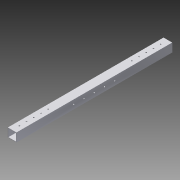
# Autodesk Inventor part: crossbar(cb)
Saved by Autodesk Inventor 2015 (Build 190159000, 159)
## iProperties
Created: 2015-10-09
Part Number: crossbar(cb)
Material: Aluminum 6061
Document SubType Name: Modeling
Designer: elilitwack
Density: 2.7 g/cm^3
Appearance: Aluminum - Flat
Mass: 205.567 g
Surface Area: 968.829 cm^2
Volume: 76.136 cm^3
RuleStatus: InUse
Author: elilitwack
Autodesk Inventor part; units mm, degrees
ref_plane "YZ Plane" through (0, 0, 0) normal (1, 0, 0) x (0, 1, 0)
ref_plane "XZ Plane" through (0, 0, 0) normal (0, 1, 0) x (-1, 0, 0)
ref_plane "XY Plane" through (0, 0, 0) normal (0, 0, 1) x (1, 0, 0)
sketch "profile_sketch" plane through (0, 0, 0) normal (0, 0, 1) x (1, 0, 0)
  line L0 (0, 0) -> (25.4, 0)
  line L1 (25.4, 0) -> (25.4, 25.4)
  line L2 (25.4, 25.4) -> (0, 25.4)
  line L3 (0, 25.4) -> (0, 0)
  line L4 (1.5875, 23.8125) -> (23.8125, 23.8125)
  line L5 (23.8125, 23.8125) -> (23.8125, 1.5875)
  line L6 (23.8125, 1.5875) -> (1.5875, 1.5875)
  line L7 (1.5875, 1.5875) -> (1.5875, 23.8125)
  dimension "d0" = 25.4
  dimension "d1" = 25.4
  dimension "d2" = 1.5875
  dimension "d3" = 1.5875
  dimension "d4" = 1.5875
  dimension "d5" = 1.5875
  constraints: 16 end point, 4 parallel, 2 horizontal, 2 perpendicular
  measures "d0" distance of L1.end L2.end
  measures "d1" distance of L0.end L1.end
  measures "d2" distance between parallel lines of L2 L4
  measures "d3" distance between parallel lines of L3 L7
  measures "d4" distance between parallel lines of L0 L6
  measures "d5" distance between parallel lines of L1 L5
extrude "profile_extrusion" add sketch "profile_sketch" along normal blind 457.2
sketch "rivet_holes_sketch" plane through (0, 25.4, 0) normal (0, 1, 0) x (1, 0, 0)
  line L0 (0, 0) -> (0, -457.2) projected
  line L1 (0, -127) -> (25.4, -127) construction
  line L2 (25.4, 0) -> (25.4, -457.2) projected
  line L3 (0, -330.2) -> (25.4, -330.2) construction
  line L4 (25.4, -457.2) -> (0, -457.2) projected
  line L5 (25.4, 0) -> (0, 0) projected
  line L6 (12.7, -457.2) -> (12.7, -436.0333) construction
  line L7 (12.7, -436.0333) -> (12.7, -414.8667) construction
  line L8 (12.7, -414.8667) -> (12.7, -393.7) construction
  line L9 (12.7, -393.7) -> (12.7, -372.5333) construction
  line L10 (12.7, -372.5333) -> (12.7, -351.3667) construction
  line L11 (12.7, -351.3667) -> (12.7, -330.2) construction
  line L12 (12.7, -127) -> (12.7, -105.8333) construction
  line L13 (12.7, -105.8333) -> (12.7, -84.6667) construction
  line L14 (12.7, -84.6667) -> (12.7, -63.5) construction
  line L15 (12.7, -63.5) -> (12.7, -42.3333) construction
  line L16 (12.7, -42.3333) -> (12.7, -21.1667) construction
  line L17 (12.7, -21.1667) -> (12.7, 0) construction
  dimension "d8" = 127
  dimension "d9" = 127
  constraints: 28 end point, 13 point on line, 10 coincident, 10 collinear, 4 midpoint, 2 vertical, 1 horizontal, 1 parallel
  measures "d8" distance between parallel lines of L4 L3
  measures "d9" distance between parallel lines of L5 L1
hole "tb_rivet_holes" at (12.7, 25.4, 105.8333) at (12.7, 25.4, 84.6667) at (12.7, 25.4, 63.5) at (12.7, 25.4, 42.3333) at (12.7, 25.4, 21.1667) at (12.7, 25.4, 351.3667) at (12.7, 25.4, 372.5333) at (12.7, 25.4, 393.7) at (12.7, 25.4, 414.8667) at (12.7, 25.4, 436.0333) direction (0, -1, 0) diameter 3.5719 depth 25.4 tip angle 118
sketch "bh_rivet_holes_sketch" plane through (25.4, 0, 0) normal (1, 0, 0) x (0, 0, -1)
  line L0 (0, 0) -> (0, 25.4) construction
  line L1 (0, 25.4) -> (-457.2, 25.4) construction
  line L2 (-457.2, 0) -> (-457.2, 25.4) construction
  line L3 (0, 0) -> (-457.2, 0) construction
  line L4 (-318.77, 12.7) -> (-288.7133, 12.7) construction
  line L5 (-288.7133, 12.7) -> (-258.6567, 12.7) construction
  line L6 (-258.6567, 12.7) -> (-228.6, 12.7) construction
  line L7 (-228.6, 12.7) -> (-198.5433, 12.7) construction
  line L8 (-198.5433, 12.7) -> (-168.4867, 12.7) construction
  line L9 (-168.4867, 12.7) -> (-138.43, 12.7) construction
  line L10 (-457.2, 0) -> (-457.2, 25.4) construction
  line L11 (-457.2, 12.7) -> (-318.77, 12.7) construction
  line L12 (-138.43, 12.7) -> (0, 12.7) construction
  line L13 (0, 23.8125) -> (0, 1.5875) construction
  point P0 (0, 0)
  dimension "d17" = 180.34
  constraints: 16 end point, 6 collinear, 5 coincident, 5 point on line, 2 horizontal, 2 midpoint
  measures "d17" distance of L9.end L4.start
hole "bh_rivet_holes" at (25.4, 12.7, 288.7133) at (25.4, 12.7, 228.6) at (25.4, 12.7, 258.6567) at (25.4, 12.7, 198.5433) at (25.4, 12.7, 168.4867) direction (-1, 0, 0) diameter 3.5719 depth 25.4 tip angle 118
sketch "pdb_ziptie_sketch" plane through (25.4, 0, 0) normal (1, 0, 0) x (0, 0, -1)
  circle A0 centre (-198.5433, 12.7) radius 1.7859 projected
  circle A1 centre (-228.6, 12.7) radius 1.7859 projected
  circle A2 centre (-288.7133, 12.7) radius 1.7859 projected
  circle A3 centre (-258.6567, 12.7) radius 1.7859 projected
  circle A4 centre (-168.4867, 12.7) radius 1.7859 projected
  line L0 (0, 0) -> (0, 25.4) projected
  line L1 (0, 25.4) -> (-457.2, 25.4) projected
  line L2 (-457.2, 0) -> (-457.2, 25.4) projected
  line L3 (0, 0) -> (-457.2, 0) projected
  line L4 (-319.7352, 9.3218) -> (-457.2, 9.3218) construction
  line L5 (-457.2, 25.4) -> (-457.2, 0) projected
  line L6 (-137.4648, 9.3218) -> (0, 9.3218) construction
  line L7 (0, 0) -> (0, 25.4) projected
  dimension "d25" = 16.0782
  dimension "d26" = 16.0782
  dimension "d27" = 182.2704
  constraints: 4 end point, 3 point on line, 1 collinear, 1 perpendicular
  measures "d25" distance from line of L1 L4.start
  measures "d26" distance from line of L1 L6.start
  measures "d27" distance of L6.start L4.start
hole "pdb_ziptie_holes" [suppressed]
equation "\"d0\" = cb_outer_diameter"
equation "\"d1\" = cb_outer_diameter"
equation "\"d2\" = cb_wall_thickness"
equation "\"d3\" = cb_wall_thickness"
equation "\"d4\" = cb_wall_thickness"
equation "\"d5\" = cb_wall_thickness"
equation "\"d6\" = cb_length"
equation "\"d8\" = tb_rivet_row_length"
equation "\"d9\" = tb_rivet_row_length"
equation "\"d10\" = rv_hole_diameter"
equation "\"d17\" = bh_length"
equation "\"d18\" = rv_hole_diameter"
equation "\"d25\" = cb_pdb_low_mount_offset"
equation "\"d26\" = cb_pdb_low_mount_offset"
equation "\"d27\" = pdb_mounting_holes_long"
equation "\"d28\" = pdb_ziptie_hole_diameter"
equation "\"cb_outer_diameter\" = 25.4"
equation "\"cb_wall_thickness\" = 1.5875"
equation "\"cb_length\" = 457.2"
equation "\"tb_rivet_row_length\" = 127"
equation "\"rv_hole_diameter\" = 3.57187"
equation "\"bh_width\" = 87.63"
equation "\"bh_length\" = 180.34"
equation "\"bh_height\" = bp_height - cb_outer_diameter"
equation "\"bh_metal_width\" = 1.5875"
equation "\"cpn_diameter\" = 69.85"
equation "\"cpn_length\" = 311.15"
equation "\"cmp_foot_seperation_long\" = 139.954"
equation "\"cmp_foot_seperation_short\" = 36.068"
equation "\"cmp_mounting_margins\" = 12.7"
equation "\"cmp_foot_bolt_diameter\" = 6.35"
equation "\"spd_fillet_size\" = 3.175"
equation "\"bp_thickness\" = 3.048"
equation "\"bp_height\" = gb_mh_seperation + st_outer_diameter"
equation "\"bp_width\" = 4 * st_rivet_distance"
equation "\"bp_axle_height\" = magic_axle_offset + gb_axle_from_edge + gb_to_bottom_of_side_assembly"
equation "\"magic_axle_offset\" = 2.286"
equation "\"bp_tensioner_width\" = 6.35"
equation "\"bp_tensioner_height\" = 50.8"
equation "\"bp_tensioner_from_bottom\" = 38.1"
equation "\"bp_tensioner_from_side\" = 25.4"
equation "\"bp_tensioner_wood_mount_from_tensioner_top\" = 12.7"
equation "\"bp_tensioner_wood_mount_diameter\" = 6.35"
equation "\"gb_mh_seperation\" = 111.1504"
equation "\"gb_mh_diameter\" = 6.35"
equation "\"gb_axle_from_edge\" = 38.1"
equation "\"gb_width\" = 127"
equation "\"gb_bearing_diameter\" = 28.575"
equation "\"gb_to_bottom_of_side_assembly\" = 4.7752"
equation "\"ncbt_rivet_row_length\" = 114.3"
equation "\"st_outer_diameter\" = 25.4"
equation "\"st_wall_thickness\" = 1.5875"
equation "\"st_length\" = 685.8"
equation "\"st_gbmh_from_center\" = 0.5 * gb_mh_seperation"
equation "\"st_cutout_depth_right\" = 203.2"
equation "\"st_cutout_depth_left\" = 203.2"
equation "\"st_rivet_distance\" = 19.05"
equation "\"so_inner_diameter\" = 7.62"
equation "\"so_wall_thickness\" = 5.08"
equation "\"so_length\" = 40.64"
equation "\"twb_width\" = st_outer_diameter"
equation "\"twb_length\" = bp_tensioner_width + 2 * twb_margin_on_each_side"
equation "\"twb_height\" = 2 * bp_tensioner_wood_mount_diameter + bp_tensioner_height + 2 * bp_tensioner_wood_mount_from_tensioner_top + twb_margin_on_each_side"
equation "\"twb_margin_on_each_side\" = 6.35"
equation "\"twb_tensioner_from_edge\" = -0.5 * bp_tensioner_height + 0.5 * twb_height"
equation "\"pdb_mounting_holes_short\" = 104.394"
equation "\"cb_pdb_low_mount_offset\" = -0.5 * pdb_mounting_holes_short + 0.5 * gb_mh_seperation + 0.5 * st_outer_diameter"
equation "\"pdb_mounting_holes_long\" = 182.2704"
equation "\"pdb_ziptie_hole_diameter\" = 6.35"
equation "\"bh_alternate_height\" = 25.4"
equation "\"bh_alternate_width\" = 81.28"
equation "\"tb_metal_thickness\" = 3.048"
equation "\"tb_hm_mounting_slot_length\" = 40.64"
equation "\"gb_mh_seperation_alt\" = 111.125"
equation "\"gb_axle_from_edge_alt\" = 43.1546"
equation "\"bp_axle_height_alt\" = magic_axle_offset + gb_axle_from_edge_alt + gb_to_bottom_of_side_assembly"
equation "\"pdb_mount_include\" = 0"
body "Solid1"
